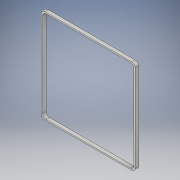
# Autodesk Inventor part: Coil1or2
Saved by Autodesk Inventor 2019 (Build 230136000, 136)
## iProperties
Created: 2021-05-17
Part Number: Coil1or2
Material: Generic
Document SubType Name: Modeling
Designer: jamieson-bl
Density: 1 g/cm^3
Appearance: Default
Author: jamieson-bl
Autodesk Inventor part; units mm, degrees
ref_plane "YZ Plane" through (0, 0, 0) normal (1, 0, 0) x (0, 1, 0)
ref_plane "XZ Plane" through (0, 0, 0) normal (0, 1, 0) x (-1, 0, 0)
ref_plane "XY Plane" through (0, 0, 0) normal (0, 0, 1) x (1, 0, 0)
sketch "Sketch1" plane through (0, 0, 0) normal (0, 0, 1) x (1, 0, 0)
  line L0 (-875, -945) -> (875, -945)
  line L1 (945, -875) -> (945, 875)
  line L2 (875, 945) -> (-875, 945)
  line L3 (-945, 875) -> (-945, -875)
  line L4 (-945, -945) -> (945, 945) construction
  line L5 (945, -945) -> (-945, 945) construction
  line L6 (-850, -920) -> (850, -920)
  line L7 (920, -850) -> (920, 850)
  line L8 (850, 920) -> (-850, 920)
  line L9 (-920, 850) -> (-920, -850)
  line L10 (-920, -920) -> (920, 920) construction
  line L11 (920, -920) -> (-920, 920) construction
  arc A0 (-850, 920) -> (-920, 850) centre (-850, 850) ccw
  arc A1 (-875, 945) -> (-945, 875) centre (-875, 875) ccw
  arc A2 (920, 850) -> (850, 920) centre (850, 850) ccw
  arc A3 (945, 875) -> (875, 945) centre (875, 875) ccw
  arc A4 (850, -920) -> (920, -850) centre (850, -850) ccw
  arc A5 (875, -945) -> (945, -875) centre (875, -875) ccw
  arc A6 (-920, -850) -> (-850, -920) centre (-850, -850) ccw
  arc A7 (-945, -875) -> (-875, -945) centre (-875, -875) ccw
  point P0 (0, 0)
  dimension "d0" = 1890
  dimension "d1" = 1890
  dimension "d2" = 1840
  dimension "d3" = 1840
  dimension "d6" = 70
  constraints: 24 end point, 16 point on circle, 16 point on line, 16 tangent, 8 centre point, 7 equal radius, 4 midpoint, 4 parallel, 2 horizontal, 2 perpendicular
  measures "d0" distance of L5.end L4.end
  measures "d1" distance of L4.end L5.start
  measures "d2" distance of L11.end L10.end
  measures "d3" distance of L10.end L11.start
  measures "d6" radius of A0
extrude "Extrusion1" add sketch "Sketch1" along normal blind 70
body "Solid1"
